Autodesk Fusion 360 part; units mm, degrees
(part 12 of 13)
move_body "Move14" bodies 13 to x (-0.996195, -0.007596, -0.086824) y (0.007596, -0.999971, 0.00033) z (-0.086824, -0.00033, 0.996224) at (0.1324, 24.9366, 0.0754)
pattern_circular "C-Pattern1" count 19 over 360 about axis through (0, 21.0013, 0) along (0, 1, 0) of bodies 11 10 12 13 makes body 14 at (9.784, 8.8123, 30.6307) makes body 15 at (19.1996, 8.8123, 25.7942) makes body 16 at (26.5347, 8.8123, 18.1625) makes body 17 at (30.9943, 8.8123, 8.5626) makes body 18 at (32.0952, 8.8123, -1.9652) makes body 19 at (30.619, 8.8187, -12.7139) makes body 20 at (24.1206, 8.8123, -21.2641) makes body 21 at (15.9092, 8.8123, -27.9439) makes body 22 at (5.9739, 8.8123, -31.5955) makes body 23 at (-4.6089, 8.8123, -31.8233) makes body 24 at (-16.9424, 10.1887, -27.2692) makes body 25 at (-23.1833, 8.8123, -22.2822) makes body 26 at (-29.1622, 8.8123, -13.5473) makes body 27 at (-31.9809, 8.8123, -3.3443) makes body 28 at (-31.334, 8.8123, 7.2211) makes body 29 at (-25.777, 10.1887, 19.1364) makes body 30 at (-18.1668, 10.1887, 26.4693) makes body 31 at (-11.0928, 8.8123, 30.1813) makes body 32 at (12.3444, 14.8255, 29.6077) makes body 33 at (21.2891, 14.8255, 23.9952) makes body 34 at (27.9268, 14.8255, 15.7825) makes body 35 at (31.5383, 14.8255, 5.8596) makes body 36 at (31.732, 14.8255, -4.6984) makes body 37 at (28.4871, 14.8255, -14.7472) makes body 38 at (22.1552, 14.8255, -23.1979) makes body 39 at (13.4224, 14.8255, -29.1348) makes body 40 at (3.2351, 14.8255, -31.9144) makes body 41 at (-7.3027, 14.8255, -31.2357) makes body 42 at (-17.0493, 14.8255, -27.172) makes body 43 at (-24.9482, 14.8255, -20.1639) makes body 44 at (-29.1662, 16.1785, -13.4098) makes body 45 at (-32.0726, 14.8255, -0.5886) makes body 46 at (-30.5259, 14.8255, 9.8572) makes body 47 at (-25.6713, 14.8255, 19.2349) makes body 48 at (-20.1593, 16.1785, 24.9818) makes body 49 at (-8.444, 14.8255, 30.9467) makes body 50 at (8.2567, 4.6533, 30.7238) makes body 51 at (17.7854, 4.6533, 26.3782) makes body 52 at (26.1953, 4.3944, 19.7024) makes body 53 at (30.237, 4.6533, 9.8921) makes body 54 at (32.7732, 4.3944, -0.5416) makes body 55 at (30.8216, 4.3944, -11.1537) makes body 56 at (24.0979, 3.4285, -21.7307) makes body 57 at (17.4719, 4.3944, -27.7329) makes body 58 at (7.3188, 3.6873, -30.6953) makes body 59 at (-3.0871, 4.6533, -31.6638) makes body 60 at (-13.2011, 4.6533, -28.9458) makes body 61 at (-21.8845, 4.6533, -23.0911) makes body 62 at (-27.9594, 3.6873, -14.6301) makes body 63 at (-31.4528, 4.6533, -4.7803) makes body 64 at (-31.9862, 3.4285, 5.8649) makes body 65 at (-27.7568, 4.6533, 15.5463) makes body 66 at (-21.205, 4.6533, 23.7166) makes body 67 at (-12.6689, 4.3944, 30.2304) makes body 68 at (9.8773, 21.2554, 30.0481) makes body 69 at (19.2453, 20.2894, 25.4259) makes body 70 at (27.2169, 20.5479, 18.3974) makes body 71 at (30.8042, 20.2894, 8.2439) makes body 72 at (31.5534, 21.2554, -2.1987) makes body 73 at (30.0454, 21.5139, -12.6328) makes body 74 at (24.5158, 20.5479, -21.8678) makes body 75 at (15.9508, 21.5139, -28.4234) makes body 76 at (5.6145, 21.2554, -31.1276) makes body 77 at (-4.8244, 20.2894, -31.5212) makes body 78 at (-15.0708, 21.5139, -28.8996) makes body 79 at (-23.8176, 20.5479, -22.6262) makes body 80 at (-29.8738, 20.5479, -13.6667) makes body 81 at (-31.7409, 20.2894, -3.0612) makes body 82 at (-31.0151, 20.2894, 7.4109) makes body 83 at (-26.7039, 21.2554, 16.9514) makes body 84 at (-20.5821, 20.5479, 25.6047) makes body 85 at (-10.7595, 20.2894, 30.0182)

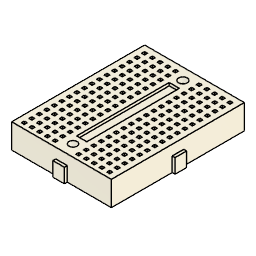
design "Mini Breadboard"
part number: 2025-09-23-19-05-31-436
Autodesk Fusion 360 part; units mm, degrees
sketch "Sketch1" plane through (0, 0, 0) normal (0, 0, 1) x (1, 0, 0)
  line L0 (17.25, 23) -> (-17.25, 23)
  line L1 (-17.25, 23) -> (-17.25, -23)
  line L2 (-17.25, -23) -> (17.25, -23)
  line L3 (17.25, -23) -> (17.25, 23)
  line L4 (17.25, 23) -> (-17.25, -23) construction
  line L5 (-17.25, 23) -> (17.25, -23) construction
  dimension "d1" = 46
  dimension "d2" = 34.5
  constraint horizontal L0
  constraint perpendicular L0 L1
  constraint parallel L0 L2
  constraint parallel L1 L3
  constraint coincident L4 origin
  constraint coincident L5 origin
  measures "d1" distance of L0.start L2.end
  measures "d2" distance of L0.start L0.end
extrude "Extrude1" add sketch "Sketch1" along normal blind 8.5
sketch "Sketch2" plane through (0, 0, 8.5) normal (0, 0, 1) x (-1, 0, 0)
  line L0 (-17.25, 23) -> (-17.25, -23)
  line L1 (-17.25, -23) -> (17.25, -23)
  line L2 (17.25, -23) -> (17.25, 23)
  line L3 (17.25, 23) -> (-17.25, 23)
  line L4 (-1.75, -16) -> (1.75, -16)
  line L5 (1.75, -16) -> (1.75, 16)
  line L6 (1.75, 16) -> (-1.75, 16)
  line L7 (-1.75, 16) -> (-1.75, -16)
  line L8 (-1.75, -16) -> (1.75, 16) construction
  line L9 (1.75, -16) -> (-1.75, 16) construction
  dimension "d5" = 32
  dimension "d6" = 3.5
  constraint horizontal L4
  constraint perpendicular L4 L5
  constraint parallel L4 L6
  constraint parallel L5 L7
  constraint coincident L8 origin
  constraint coincident L9 origin
  measures "d5" distance of L4.start L6.end
  measures "d6" distance of L4.start L4.end
extrude "Extrude2" cut sketch "Sketch2" against normal blind 1 contours L4 L5 L6 L7
sketch "Sketch3" plane through (0, 0, 8.5) normal (0, 0, 1) x (-1, 0, 0)
  line L0 (1.75, -16) -> (-1.75, -16)
  line L1 (-1.75, -16) -> (-1.75, 16)
  line L2 (-1.75, 16) -> (1.75, 16)
  line L3 (1.75, 16) -> (1.75, -16)
  line L4 (-17.25, 23) -> (-17.25, -23)
  line L5 (-17.25, -23) -> (17.25, -23)
  line L6 (17.25, -23) -> (17.25, 23)
  line L7 (17.25, 23) -> (-17.25, 23)
  line L8 (15.25, -20) -> (14.25, -20)
  line L9 (14.25, -20) -> (14.25, -21)
  line L10 (14.25, -21) -> (15.25, -21)
  line L11 (15.25, -21) -> (15.25, -20)
  line L12 (15.25, -20) -> (14.25, -21) construction
  line L13 (14.25, -20) -> (15.25, -21) construction
  point P0 (14.75, -20.5)
  dimension "d9" = 1
  dimension "d10" = 1
  dimension "d11" = 2
  dimension "d12" = 2
  constraint horizontal L8
  constraint perpendicular L8 L9
  constraint parallel L8 L10
  constraint parallel L9 L11
  constraint coincident L12 P0
  constraint coincident L13 P0
  measures "d9" distance of L9.end L10.end
  measures "d10" distance of L8.end L9.end
  measures "d11" distance of L6 L11
  measures "d12" distance of L5 L10
extrude "Extrude3" cut sketch "Sketch3" against normal blind 1 contours L8 L9 L10 L11
pattern_linear "R-Pattern1" count 5 spacing 2.67 along (1, 0, 0) count 17 spacing 2.6 along (0, -1, 0) of "Extrude3"
sketch "Sketch4" plane through (0, 0, 8.5) normal (0, 0, 1) x (-1, 0, 0)
  line L0 (3.57, 21.6) -> (4.57, 21.6)
  line L1 (4.57, 21.6) -> (4.57, 20.6)
  line L2 (4.57, 20.6) -> (3.57, 20.6)
  line L3 (3.57, 20.6) -> (3.57, 21.6)
  line L4 (6.24, 21.6) -> (7.24, 21.6)
  line L5 (7.24, 21.6) -> (7.24, 20.6)
  line L6 (7.24, 20.6) -> (6.24, 20.6)
  line L7 (6.24, 20.6) -> (6.24, 21.6)
  line L8 (8.91, 21.6) -> (9.91, 21.6)
  line L9 (9.91, 21.6) -> (9.91, 20.6)
  line L10 (9.91, 20.6) -> (8.91, 20.6)
  line L11 (8.91, 20.6) -> (8.91, 21.6)
  line L12 (11.58, 21.6) -> (12.58, 21.6)
  line L13 (12.58, 21.6) -> (12.58, 20.6)
  line L14 (12.58, 20.6) -> (11.58, 20.6)
  line L15 (11.58, 20.6) -> (11.58, 21.6)
  line L16 (14.25, 21.6) -> (15.25, 21.6)
  line L17 (15.25, 21.6) -> (15.25, 20.6)
  line L18 (15.25, 20.6) -> (14.25, 20.6)
  line L19 (14.25, 20.6) -> (14.25, 21.6)
  line L20 (3.57, 19) -> (4.57, 19)
  line L21 (4.57, 19) -> (4.57, 18)
  line L22 (4.57, 18) -> (3.57, 18)
  line L23 (3.57, 18) -> (3.57, 19)
  line L24 (6.24, 19) -> (7.24, 19)
  line L25 (7.24, 19) -> (7.24, 18)
  line L26 (7.24, 18) -> (6.24, 18)
  line L27 (6.24, 18) -> (6.24, 19)
  line L28 (8.91, 19) -> (9.91, 19)
  line L29 (9.91, 19) -> (9.91, 18)
  line L30 (9.91, 18) -> (8.91, 18)
  line L31 (8.91, 18) -> (8.91, 19)
  line L32 (11.58, 19) -> (12.58, 19)
  line L33 (12.58, 19) -> (12.58, 18)
  line L34 (12.58, 18) -> (11.58, 18)
  line L35 (11.58, 18) -> (11.58, 19)
  line L36 (14.25, 19) -> (15.25, 19)
  line L37 (15.25, 19) -> (15.25, 18)
  line L38 (15.25, 18) -> (14.25, 18)
  line L39 (14.25, 18) -> (14.25, 19)
  line L40 (3.57, 16.4) -> (4.57, 16.4)
  line L41 (4.57, 16.4) -> (4.57, 15.4)
  line L42 (4.57, 15.4) -> (3.57, 15.4)
  line L43 (3.57, 15.4) -> (3.57, 16.4)
  line L44 (6.24, 16.4) -> (7.24, 16.4)
  line L45 (7.24, 16.4) -> (7.24, 15.4)
  line L46 (7.24, 15.4) -> (6.24, 15.4)
  line L47 (6.24, 15.4) -> (6.24, 16.4)
  line L48 (8.91, 16.4) -> (9.91, 16.4)
  line L49 (9.91, 16.4) -> (9.91, 15.4)
  line L50 (9.91, 15.4) -> (8.91, 15.4)
  line L51 (8.91, 15.4) -> (8.91, 16.4)
  line L52 (11.58, 16.4) -> (12.58, 16.4)
  line L53 (12.58, 16.4) -> (12.58, 15.4)
  line L54 (12.58, 15.4) -> (11.58, 15.4)
  line L55 (11.58, 15.4) -> (11.58, 16.4)
  line L56 (14.25, 16.4) -> (15.25, 16.4)
  line L57 (15.25, 16.4) -> (15.25, 15.4)
  line L58 (15.25, 15.4) -> (14.25, 15.4)
  line L59 (14.25, 15.4) -> (14.25, 16.4)
  line L60 (3.57, 13.8) -> (4.57, 13.8)
  line L61 (4.57, 13.8) -> (4.57, 12.8)
  line L62 (4.57, 12.8) -> (3.57, 12.8)
  line L63 (3.57, 12.8) -> (3.57, 13.8)
  line L64 (6.24, 13.8) -> (7.24, 13.8)
  line L65 (7.24, 13.8) -> (7.24, 12.8)
  line L66 (7.24, 12.8) -> (6.24, 12.8)
  line L67 (6.24, 12.8) -> (6.24, 13.8)
  line L68 (8.91, 13.8) -> (9.91, 13.8)
  line L69 (9.91, 13.8) -> (9.91, 12.8)
  line L70 (9.91, 12.8) -> (8.91, 12.8)
  line L71 (8.91, 12.8) -> (8.91, 13.8)
  line L72 (11.58, 13.8) -> (12.58, 13.8)
  line L73 (12.58, 13.8) -> (12.58, 12.8)
  line L74 (12.58, 12.8) -> (11.58, 12.8)
  line L75 (11.58, 12.8) -> (11.58, 13.8)
  line L76 (14.25, 13.8) -> (15.25, 13.8)
  line L77 (15.25, 13.8) -> (15.25, 12.8)
  line L78 (15.25, 12.8) -> (14.25, 12.8)
  line L79 (14.25, 12.8) -> (14.25, 13.8)
  line L80 (3.57, 11.2) -> (4.57, 11.2)
  line L81 (4.57, 11.2) -> (4.57, 10.2)
  line L82 (4.57, 10.2) -> (3.57, 10.2)
  line L83 (3.57, 10.2) -> (3.57, 11.2)
  line L84 (6.24, 11.2) -> (7.24, 11.2)
  line L85 (7.24, 11.2) -> (7.24, 10.2)
  line L86 (7.24, 10.2) -> (6.24, 10.2)
  line L87 (6.24, 10.2) -> (6.24, 11.2)
  line L88 (8.91, 11.2) -> (9.91, 11.2)
  line L89 (9.91, 11.2) -> (9.91, 10.2)
  line L90 (9.91, 10.2) -> (8.91, 10.2)
  line L91 (8.91, 10.2) -> (8.91, 11.2)
  line L92 (11.58, 11.2) -> (12.58, 11.2)
  line L93 (12.58, 11.2) -> (12.58, 10.2)
  line L94 (12.58, 10.2) -> (11.58, 10.2)
  line L95 (11.58, 10.2) -> (11.58, 11.2)
  line L96 (14.25, 11.2) -> (15.25, 11.2)
  line L97 (15.25, 11.2) -> (15.25, 10.2)
  line L98 (15.25, 10.2) -> (14.25, 10.2)
  line L99 (14.25, 10.2) -> (14.25, 11.2)
  line L100 (3.57, 8.6) -> (4.57, 8.6)
  line L101 (4.57, 8.6) -> (4.57, 7.6)
  line L102 (4.57, 7.6) -> (3.57, 7.6)
  line L103 (3.57, 7.6) -> (3.57, 8.6)
  line L104 (6.24, 8.6) -> (7.24, 8.6)
  line L105 (7.24, 8.6) -> (7.24, 7.6)
  line L106 (7.24, 7.6) -> (6.24, 7.6)
  line L107 (6.24, 7.6) -> (6.24, 8.6)
  line L108 (8.91, 8.6) -> (9.91, 8.6)
  line L109 (9.91, 8.6) -> (9.91, 7.6)
  line L110 (9.91, 7.6) -> (8.91, 7.6)
  line L111 (8.91, 7.6) -> (8.91, 8.6)
  line L112 (11.58, 8.6) -> (12.58, 8.6)
  line L113 (12.58, 8.6) -> (12.58, 7.6)
  line L114 (12.58, 7.6) -> (11.58, 7.6)
  line L115 (11.58, 7.6) -> (11.58, 8.6)
  line L116 (14.25, 8.6) -> (15.25, 8.6)
  line L117 (15.25, 8.6) -> (15.25, 7.6)
  line L118 (15.25, 7.6) -> (14.25, 7.6)
  line L119 (14.25, 7.6) -> (14.25, 8.6)
  line L120 (3.57, 6) -> (4.57, 6)
  line L121 (4.57, 6) -> (4.57, 5)
  line L122 (4.57, 5) -> (3.57, 5)
  line L123 (3.57, 5) -> (3.57, 6)
  line L124 (6.24, 6) -> (7.24, 6)
  line L125 (7.24, 6) -> (7.24, 5)
  line L126 (7.24, 5) -> (6.24, 5)
  line L127 (6.24, 5) -> (6.24, 6)
  line L128 (8.91, 6) -> (9.91, 6)
  line L129 (9.91, 6) -> (9.91, 5)
  line L130 (9.91, 5) -> (8.91, 5)
  line L131 (8.91, 5) -> (8.91, 6)
  line L132 (11.58, 6) -> (12.58, 6)
  line L133 (12.58, 6) -> (12.58, 5)
  line L134 (12.58, 5) -> (11.58, 5)
  line L135 (11.58, 5) -> (11.58, 6)
  line L136 (14.25, 6) -> (15.25, 6)
  line L137 (15.25, 6) -> (15.25, 5)
  line L138 (15.25, 5) -> (14.25, 5)
  line L139 (14.25, 5) -> (14.25, 6)
  line L140 (3.57, 3.4) -> (4.57, 3.4)
  line L141 (4.57, 3.4) -> (4.57, 2.4)
  line L142 (4.57, 2.4) -> (3.57, 2.4)
  line L143 (3.57, 2.4) -> (3.57, 3.4)
  line L144 (6.24, 3.4) -> (7.24, 3.4)
  line L145 (7.24, 3.4) -> (7.24, 2.4)
  line L146 (7.24, 2.4) -> (6.24, 2.4)
  line L147 (6.24, 2.4) -> (6.24, 3.4)
  line L148 (8.91, 3.4) -> (9.91, 3.4)
  line L149 (9.91, 3.4) -> (9.91, 2.4)
  line L150 (9.91, 2.4) -> (8.91, 2.4)
  line L151 (8.91, 2.4) -> (8.91, 3.4)
  line L152 (11.58, 3.4) -> (12.58, 3.4)
  line L153 (12.58, 3.4) -> (12.58, 2.4)
  line L154 (12.58, 2.4) -> (11.58, 2.4)
  line L155 (11.58, 2.4) -> (11.58, 3.4)
  line L156 (14.25, 3.4) -> (15.25, 3.4)
  line L157 (15.25, 3.4) -> (15.25, 2.4)
  line L158 (15.25, 2.4) -> (14.25, 2.4)
  line L159 (14.25, 2.4) -> (14.25, 3.4)
  line L160 (3.57, 0.8) -> (4.57, 0.8)
  line L161 (4.57, 0.8) -> (4.57, -0.2)
  line L162 (4.57, -0.2) -> (3.57, -0.2)
  line L163 (3.57, -0.2) -> (3.57, 0.8)
  line L164 (6.24, 0.8) -> (7.24, 0.8)
  line L165 (7.24, 0.8) -> (7.24, -0.2)
  line L166 (7.24, -0.2) -> (6.24, -0.2)
  line L167 (6.24, -0.2) -> (6.24, 0.8)
  line L168 (8.91, 0.8) -> (9.91, 0.8)
  line L169 (9.91, 0.8) -> (9.91, -0.2)
  line L170 (9.91, -0.2) -> (8.91, -0.2)
  line L171 (8.91, -0.2) -> (8.91, 0.8)
  line L172 (11.58, 0.8) -> (12.58, 0.8)
  line L173 (12.58, 0.8) -> (12.58, -0.2)
  line L174 (12.58, -0.2) -> (11.58, -0.2)
  line L175 (11.58, -0.2) -> (11.58, 0.8)
  line L176 (14.25, 0.8) -> (15.25, 0.8)
  line L177 (15.25, 0.8) -> (15.25, -0.2)
  line L178 (15.25, -0.2) -> (14.25, -0.2)
  line L179 (14.25, -0.2) -> (14.25, 0.8)
  line L180 (3.57, -1.8) -> (4.57, -1.8)
  line L181 (4.57, -1.8) -> (4.57, -2.8)
  line L182 (4.57, -2.8) -> (3.57, -2.8)
  line L183 (3.57, -2.8) -> (3.57, -1.8)
  line L184 (6.24, -1.8) -> (7.24, -1.8)
  line L185 (7.24, -1.8) -> (7.24, -2.8)
  line L186 (7.24, -2.8) -> (6.24, -2.8)
  line L187 (6.24, -2.8) -> (6.24, -1.8)
  line L188 (8.91, -1.8) -> (9.91, -1.8)
  line L189 (9.91, -1.8) -> (9.91, -2.8)
  line L190 (9.91, -2.8) -> (8.91, -2.8)
  line L191 (8.91, -2.8) -> (8.91, -1.8)
  line L192 (11.58, -1.8) -> (12.58, -1.8)
  line L193 (12.58, -1.8) -> (12.58, -2.8)
  line L194 (12.58, -2.8) -> (11.58, -2.8)
  line L195 (11.58, -2.8) -> (11.58, -1.8)
  line L196 (14.25, -1.8) -> (15.25, -1.8)
  line L197 (15.25, -1.8) -> (15.25, -2.8)
  line L198 (15.25, -2.8) -> (14.25, -2.8)
  line L199 (14.25, -2.8) -> (14.25, -1.8)
  line L200 (3.57, -4.4) -> (4.57, -4.4)
  line L201 (4.57, -4.4) -> (4.57, -5.4)
  line L202 (4.57, -5.4) -> (3.57, -5.4)
  line L203 (3.57, -5.4) -> (3.57, -4.4)
  line L204 (6.24, -4.4) -> (7.24, -4.4)
  line L205 (7.24, -4.4) -> (7.24, -5.4)
  line L206 (7.24, -5.4) -> (6.24, -5.4)
  line L207 (6.24, -5.4) -> (6.24, -4.4)
  line L208 (8.91, -4.4) -> (9.91, -4.4)
  line L209 (9.91, -4.4) -> (9.91, -5.4)
  line L210 (9.91, -5.4) -> (8.91, -5.4)
  line L211 (8.91, -5.4) -> (8.91, -4.4)
  line L212 (11.58, -4.4) -> (12.58, -4.4)
  line L213 (12.58, -4.4) -> (12.58, -5.4)
  line L214 (12.58, -5.4) -> (11.58, -5.4)
  line L215 (11.58, -5.4) -> (11.58, -4.4)
  line L216 (14.25, -4.4) -> (15.25, -4.4)
  line L217 (15.25, -4.4) -> (15.25, -5.4)
  line L218 (15.25, -5.4) -> (14.25, -5.4)
  line L219 (14.25, -5.4) -> (14.25, -4.4)
  line L220 (3.57, -7) -> (4.57, -7)
  line L221 (4.57, -7) -> (4.57, -8)
  line L222 (4.57, -8) -> (3.57, -8)
  line L223 (3.57, -8) -> (3.57, -7)
  line L224 (6.24, -7) -> (7.24, -7)
  line L225 (7.24, -7) -> (7.24, -8)
  line L226 (7.24, -8) -> (6.24, -8)
  line L227 (6.24, -8) -> (6.24, -7)
  line L228 (8.91, -7) -> (9.91, -7)
  line L229 (9.91, -7) -> (9.91, -8)
  line L230 (9.91, -8) -> (8.91, -8)
  line L231 (8.91, -8) -> (8.91, -7)
  line L232 (11.58, -7) -> (12.58, -7)
  line L233 (12.58, -7) -> (12.58, -8)
  line L234 (12.58, -8) -> (11.58, -8)
  line L235 (11.58, -8) -> (11.58, -7)
  line L236 (14.25, -7) -> (15.25, -7)
  line L237 (15.25, -7) -> (15.25, -8)
  line L238 (15.25, -8) -> (14.25, -8)
  line L239 (14.25, -8) -> (14.25, -7)
  line L240 (3.57, -9.6) -> (4.57, -9.6)
  line L241 (4.57, -9.6) -> (4.57, -10.6)
  line L242 (4.57, -10.6) -> (3.57, -10.6)
  line L243 (3.57, -10.6) -> (3.57, -9.6)
  line L244 (6.24, -9.6) -> (7.24, -9.6)
  line L245 (7.24, -9.6) -> (7.24, -10.6)
  line L246 (7.24, -10.6) -> (6.24, -10.6)
  line L247 (6.24, -10.6) -> (6.24, -9.6)
  line L248 (8.91, -9.6) -> (9.91, -9.6)
  line L249 (9.91, -9.6) -> (9.91, -10.6)
  line L250 (9.91, -10.6) -> (8.91, -10.6)
  line L251 (8.91, -10.6) -> (8.91, -9.6)
  line L252 (11.58, -9.6) -> (12.58, -9.6)
  line L253 (12.58, -9.6) -> (12.58, -10.6)
  line L254 (12.58, -10.6) -> (11.58, -10.6)
  line L255 (11.58, -10.6) -> (11.58, -9.6)
  line L256 (14.25, -9.6) -> (15.25, -9.6)
  line L257 (15.25, -9.6) -> (15.25, -10.6)
  line L258 (15.25, -10.6) -> (14.25, -10.6)
  line L259 (14.25, -10.6) -> (14.25, -9.6)
  line L260 (3.57, -12.2) -> (4.57, -12.2)
  line L261 (4.57, -12.2) -> (4.57, -13.2)
  line L262 (4.57, -13.2) -> (3.57, -13.2)
  line L263 (3.57, -13.2) -> (3.57, -12.2)
  line L264 (6.24, -12.2) -> (7.24, -12.2)
  line L265 (7.24, -12.2) -> (7.24, -13.2)
  line L266 (7.24, -13.2) -> (6.24, -13.2)
  line L267 (6.24, -13.2) -> (6.24, -12.2)
  line L268 (8.91, -12.2) -> (9.91, -12.2)
  line L269 (9.91, -12.2) -> (9.91, -13.2)
  line L270 (9.91, -13.2) -> (8.91, -13.2)
  line L271 (8.91, -13.2) -> (8.91, -12.2)
  line L272 (11.58, -12.2) -> (12.58, -12.2)
  line L273 (12.58, -12.2) -> (12.58, -13.2)
  line L274 (12.58, -13.2) -> (11.58, -13.2)
  line L275 (11.58, -13.2) -> (11.58, -12.2)
  line L276 (14.25, -12.2) -> (15.25, -12.2)
  line L277 (15.25, -12.2) -> (15.25, -13.2)
  line L278 (15.25, -13.2) -> (14.25, -13.2)
  line L279 (14.25, -13.2) -> (14.25, -12.2)
  line L280 (3.57, -14.8) -> (4.57, -14.8)
  line L281 (4.57, -14.8) -> (4.57, -15.8)
  line L282 (4.57, -15.8) -> (3.57, -15.8)
  line L283 (3.57, -15.8) -> (3.57, -14.8)
  line L284 (6.24, -14.8) -> (7.24, -14.8)
  line L285 (7.24, -14.8) -> (7.24, -15.8)
  line L286 (7.24, -15.8) -> (6.24, -15.8)
  line L287 (6.24, -15.8) -> (6.24, -14.8)
  line L288 (8.91, -14.8) -> (9.91, -14.8)
  line L289 (9.91, -14.8) -> (9.91, -15.8)
  line L290 (9.91, -15.8) -> (8.91, -15.8)
  line L291 (8.91, -15.8) -> (8.91, -14.8)
  line L292 (11.58, -14.8) -> (12.58, -14.8)
  line L293 (12.58, -14.8) -> (12.58, -15.8)
  line L294 (12.58, -15.8) -> (11.58, -15.8)
  line L295 (11.58, -15.8) -> (11.58, -14.8)
  line L296 (14.25, -14.8) -> (15.25, -14.8)
  line L297 (15.25, -14.8) -> (15.25, -15.8)
  line L298 (15.25, -15.8) -> (14.25, -15.8)
  line L299 (14.25, -15.8) -> (14.25, -14.8)
  line L300 (3.57, -17.4) -> (4.57, -17.4)
  line L301 (4.57, -17.4) -> (4.57, -18.4)
  line L302 (4.57, -18.4) -> (3.57, -18.4)
  line L303 (3.57, -18.4) -> (3.57, -17.4)
  line L304 (6.24, -17.4) -> (7.24, -17.4)
  line L305 (7.24, -17.4) -> (7.24, -18.4)
  line L306 (7.24, -18.4) -> (6.24, -18.4)
  line L307 (6.24, -18.4) -> (6.24, -17.4)
  line L308 (8.91, -17.4) -> (9.91, -17.4)
  line L309 (9.91, -17.4) -> (9.91, -18.4)
  line L310 (9.91, -18.4) -> (8.91, -18.4)
  line L311 (8.91, -18.4) -> (8.91, -17.4)
  line L312 (11.58, -17.4) -> (12.58, -17.4)
  line L313 (12.58, -17.4) -> (12.58, -18.4)
  line L314 (12.58, -18.4) -> (11.58, -18.4)
  line L315 (11.58, -18.4) -> (11.58, -17.4)
  line L316 (14.25, -17.4) -> (15.25, -17.4)
  line L317 (15.25, -17.4) -> (15.25, -18.4)
  line L318 (15.25, -18.4) -> (14.25, -18.4)
  line L319 (14.25, -18.4) -> (14.25, -17.4)
  line L320 (3.57, -20) -> (4.57, -20)
  line L321 (4.57, -20) -> (4.57, -21)
  line L322 (4.57, -21) -> (3.57, -21)
  line L323 (3.57, -21) -> (3.57, -20)
  line L324 (6.24, -20) -> (7.24, -20)
  line L325 (7.24, -20) -> (7.24, -21)
  line L326 (7.24, -21) -> (6.24, -21)
  line L327 (6.24, -21) -> (6.24, -20)
  line L328 (8.91, -20) -> (9.91, -20)
  line L329 (9.91, -20) -> (9.91, -21)
  line L330 (9.91, -21) -> (8.91, -21)
  line L331 (8.91, -21) -> (8.91, -20)
  line L332 (11.58, -20) -> (12.58, -20)
  line L333 (12.58, -20) -> (12.58, -21)
  line L334 (12.58, -21) -> (11.58, -21)
  line L335 (11.58, -21) -> (11.58, -20)
  line L336 (14.25, -20) -> (15.25, -20)
  line L337 (15.25, -20) -> (15.25, -21)
  line L338 (15.25, -21) -> (14.25, -21)
  line L339 (14.25, -21) -> (14.25, -20)
  line L340 (1.75, -16) -> (-1.75, -16)
  line L341 (-1.75, -16) -> (-1.75, 16)
  line L342 (-1.75, 16) -> (1.75, 16)
  line L343 (1.75, 16) -> (1.75, -16)
  line L344 (-17.25, 23) -> (-17.25, -23)
  line L345 (-17.25, -23) -> (17.25, -23)
  line L346 (17.25, -23) -> (17.25, 23)
  line L347 (17.25, 23) -> (-17.25, 23)
  line L348 (-14.25, -20) -> (-15.25, -20)
  line L349 (-15.25, -20) -> (-15.25, -21)
  line L350 (-15.25, -21) -> (-14.25, -21)
  line L351 (-14.25, -21) -> (-14.25, -20)
  line L352 (-14.25, -20) -> (-15.25, -21) construction
  line L353 (-15.25, -20) -> (-14.25, -21) construction
  point P0 (-14.75, -20.5)
  dimension "d19" = 1
  dimension "d20" = 1
  dimension "d21" = 2
  dimension "d22" = 2
  constraint horizontal L348
  constraint perpendicular L348 L349
  constraint parallel L348 L350
  constraint parallel L349 L351
  constraint coincident L352 P0
  constraint coincident L353 P0
  measures "d19" distance of L348.start L348.end
  measures "d20" distance of L348.end L349.end
  measures "d21" distance of L344 L349
  measures "d22" distance of L345 L350
extrude "Extrude4" cut sketch "Sketch4" against normal blind 1 contours L348 L349 L350 L351
pattern_linear "R-Pattern2" count 5 spacing 2.67 along (-1, 0, 0) count 17 spacing 2.6 along (0, -1, 0) of "Extrude4"
sketch "Sketch5" plane through (0, 0, 8.5) normal (0, 0, 1) x (-1, 0, 0)
  line L0 (-4.57, 21.6) -> (-3.57, 21.6)
  line L1 (-3.57, 21.6) -> (-3.57, 20.6)
  line L2 (-3.57, 20.6) -> (-4.57, 20.6)
  line L3 (-4.57, 20.6) -> (-4.57, 21.6)
  line L4 (-7.24, 21.6) -> (-6.24, 21.6)
  line L5 (-6.24, 21.6) -> (-6.24, 20.6)
  line L6 (-6.24, 20.6) -> (-7.24, 20.6)
  line L7 (-7.24, 20.6) -> (-7.24, 21.6)
  line L8 (-9.91, 21.6) -> (-8.91, 21.6)
  line L9 (-8.91, 21.6) -> (-8.91, 20.6)
  line L10 (-8.91, 20.6) -> (-9.91, 20.6)
  line L11 (-9.91, 20.6) -> (-9.91, 21.6)
  line L12 (-12.58, 21.6) -> (-11.58, 21.6)
  line L13 (-11.58, 21.6) -> (-11.58, 20.6)
  line L14 (-11.58, 20.6) -> (-12.58, 20.6)
  line L15 (-12.58, 20.6) -> (-12.58, 21.6)
  line L16 (-15.25, 21.6) -> (-14.25, 21.6)
  line L17 (-14.25, 21.6) -> (-14.25, 20.6)
  line L18 (-14.25, 20.6) -> (-15.25, 20.6)
  line L19 (-15.25, 20.6) -> (-15.25, 21.6)
  line L20 (-4.57, 19) -> (-3.57, 19)
  line L21 (-3.57, 19) -> (-3.57, 18)
  line L22 (-3.57, 18) -> (-4.57, 18)
  line L23 (-4.57, 18) -> (-4.57, 19)
  line L24 (-7.24, 19) -> (-6.24, 19)
  line L25 (-6.24, 19) -> (-6.24, 18)
  line L26 (-6.24, 18) -> (-7.24, 18)
  line L27 (-7.24, 18) -> (-7.24, 19)
  line L28 (-9.91, 19) -> (-8.91, 19)
  line L29 (-8.91, 19) -> (-8.91, 18)
  line L30 (-8.91, 18) -> (-9.91, 18)
  line L31 (-9.91, 18) -> (-9.91, 19)
  line L32 (-12.58, 19) -> (-11.58, 19)
  line L33 (-11.58, 19) -> (-11.58, 18)
  line L34 (-11.58, 18) -> (-12.58, 18)
  line L35 (-12.58, 18) -> (-12.58, 19)
  line L36 (-15.25, 19) -> (-14.25, 19)
  line L37 (-14.25, 19) -> (-14.25, 18)
  line L38 (-14.25, 18) -> (-15.25, 18)
  line L39 (-15.25, 18) -> (-15.25, 19)
  line L40 (-4.57, 16.4) -> (-3.57, 16.4)
  line L41 (-3.57, 16.4) -> (-3.57, 15.4)
  line L42 (-3.57, 15.4) -> (-4.57, 15.4)
  line L43 (-4.57, 15.4) -> (-4.57, 16.4)
  line L44 (-7.24, 16.4) -> (-6.24, 16.4)
  line L45 (-6.24, 16.4) -> (-6.24, 15.4)
  line L46 (-6.24, 15.4) -> (-7.24, 15.4)
  line L47 (-7.24, 15.4) -> (-7.24, 16.4)
  line L48 (-9.91, 16.4) -> (-8.91, 16.4)
  line L49 (-8.91, 16.4) -> (-8.91, 15.4)
  line L50 (-8.91, 15.4) -> (-9.91, 15.4)
  line L51 (-9.91, 15.4) -> (-9.91, 16.4)
  line L52 (-12.58, 16.4) -> (-11.58, 16.4)
  line L53 (-11.58, 16.4) -> (-11.58, 15.4)
  line L54 (-11.58, 15.4) -> (-12.58, 15.4)
  line L55 (-12.58, 15.4) -> (-12.58, 16.4)
  line L56 (-15.25, 16.4) -> (-14.25, 16.4)
  line L57 (-14.25, 16.4) -> (-14.25, 15.4)
  line L58 (-14.25, 15.4) -> (-15.25, 15.4)
  line L59 (-15.25, 15.4) -> (-15.25, 16.4)
  line L60 (-4.57, 13.8) -> (-3.57, 13.8)
  line L61 (-3.57, 13.8) -> (-3.57, 12.8)
  line L62 (-3.57, 12.8) -> (-4.57, 12.8)
  line L63 (-4.57, 12.8) -> (-4.57, 13.8)
  line L64 (-7.24, 13.8) -> (-6.24, 13.8)
  line L65 (-6.24, 13.8) -> (-6.24, 12.8)
  line L66 (-6.24, 12.8) -> (-7.24, 12.8)
  line L67 (-7.24, 12.8) -> (-7.24, 13.8)
  line L68 (-9.91, 13.8) -> (-8.91, 13.8)
  line L69 (-8.91, 13.8) -> (-8.91, 12.8)
  line L70 (-8.91, 12.8) -> (-9.91, 12.8)
  line L71 (-9.91, 12.8) -> (-9.91, 13.8)
  line L72 (-12.58, 13.8) -> (-11.58, 13.8)
  line L73 (-11.58, 13.8) -> (-11.58, 12.8)
  line L74 (-11.58, 12.8) -> (-12.58, 12.8)
  line L75 (-12.58, 12.8) -> (-12.58, 13.8)
  line L76 (-15.25, 13.8) -> (-14.25, 13.8)
  line L77 (-14.25, 13.8) -> (-14.25, 12.8)
  line L78 (-14.25, 12.8) -> (-15.25, 12.8)
  line L79 (-15.25, 12.8) -> (-15.25, 13.8)
  line L80 (-4.57, 11.2) -> (-3.57, 11.2)
  line L81 (-3.57, 11.2) -> (-3.57, 10.2)
  line L82 (-3.57, 10.2) -> (-4.57, 10.2)
  line L83 (-4.57, 10.2) -> (-4.57, 11.2)
  line L84 (-7.24, 11.2) -> (-6.24, 11.2)
  line L85 (-6.24, 11.2) -> (-6.24, 10.2)
  line L86 (-6.24, 10.2) -> (-7.24, 10.2)
  line L87 (-7.24, 10.2) -> (-7.24, 11.2)
  line L88 (-9.91, 11.2) -> (-8.91, 11.2)
  line L89 (-8.91, 11.2) -> (-8.91, 10.2)
  line L90 (-8.91, 10.2) -> (-9.91, 10.2)
  line L91 (-9.91, 10.2) -> (-9.91, 11.2)
  line L92 (-12.58, 11.2) -> (-11.58, 11.2)
  line L93 (-11.58, 11.2) -> (-11.58, 10.2)
  line L94 (-11.58, 10.2) -> (-12.58, 10.2)
  line L95 (-12.58, 10.2) -> (-12.58, 11.2)
  line L96 (-15.25, 11.2) -> (-14.25, 11.2)
  line L97 (-14.25, 11.2) -> (-14.25, 10.2)
  line L98 (-14.25, 10.2) -> (-15.25, 10.2)
  line L99 (-15.25, 10.2) -> (-15.25, 11.2)
  line L100 (-4.57, 8.6) -> (-3.57, 8.6)
  line L101 (-3.57, 8.6) -> (-3.57, 7.6)
  line L102 (-3.57, 7.6) -> (-4.57, 7.6)
  line L103 (-4.57, 7.6) -> (-4.57, 8.6)
  line L104 (-7.24, 8.6) -> (-6.24, 8.6)
  line L105 (-6.24, 8.6) -> (-6.24, 7.6)
  line L106 (-6.24, 7.6) -> (-7.24, 7.6)
  line L107 (-7.24, 7.6) -> (-7.24, 8.6)
  line L108 (-9.91, 8.6) -> (-8.91, 8.6)
  line L109 (-8.91, 8.6) -> (-8.91, 7.6)
  line L110 (-8.91, 7.6) -> (-9.91, 7.6)
  line L111 (-9.91, 7.6) -> (-9.91, 8.6)
  line L112 (-12.58, 8.6) -> (-11.58, 8.6)
  line L113 (-11.58, 8.6) -> (-11.58, 7.6)
  line L114 (-11.58, 7.6) -> (-12.58, 7.6)
  line L115 (-12.58, 7.6) -> (-12.58, 8.6)
  line L116 (-15.25, 8.6) -> (-14.25, 8.6)
  line L117 (-14.25, 8.6) -> (-14.25, 7.6)
  line L118 (-14.25, 7.6) -> (-15.25, 7.6)
  line L119 (-15.25, 7.6) -> (-15.25, 8.6)
  line L120 (-4.57, 6) -> (-3.57, 6)
  line L121 (-3.57, 6) -> (-3.57, 5)
  line L122 (-3.57, 5) -> (-4.57, 5)
  line L123 (-4.57, 5) -> (-4.57, 6)
  line L124 (-7.24, 6) -> (-6.24, 6)
  line L125 (-6.24, 6) -> (-6.24, 5)
  line L126 (-6.24, 5) -> (-7.24, 5)
  line L127 (-7.24, 5) -> (-7.24, 6)
  line L128 (-9.91, 6) -> (-8.91, 6)
  line L129 (-8.91, 6) -> (-8.91, 5)
  line L130 (-8.91, 5) -> (-9.91, 5)
  line L131 (-9.91, 5) -> (-9.91, 6)
  line L132 (-12.58, 6) -> (-11.58, 6)
  line L133 (-11.58, 6) -> (-11.58, 5)
  line L134 (-11.58, 5) -> (-12.58, 5)
  line L135 (-12.58, 5) -> (-12.58, 6)
  line L136 (-15.25, 6) -> (-14.25, 6)
  line L137 (-14.25, 6) -> (-14.25, 5)
  line L138 (-14.25, 5) -> (-15.25, 5)
  line L139 (-15.25, 5) -> (-15.25, 6)
  line L140 (-4.57, 3.4) -> (-3.57, 3.4)
  line L141 (-3.57, 3.4) -> (-3.57, 2.4)
  line L142 (-3.57, 2.4) -> (-4.57, 2.4)
  line L143 (-4.57, 2.4) -> (-4.57, 3.4)
  line L144 (-7.24, 3.4) -> (-6.24, 3.4)
  line L145 (-6.24, 3.4) -> (-6.24, 2.4)
  line L146 (-6.24, 2.4) -> (-7.24, 2.4)
  line L147 (-7.24, 2.4) -> (-7.24, 3.4)
  line L148 (-9.91, 3.4) -> (-8.91, 3.4)
  line L149 (-8.91, 3.4) -> (-8.91, 2.4)
  line L150 (-8.91, 2.4) -> (-9.91, 2.4)
  line L151 (-9.91, 2.4) -> (-9.91, 3.4)
  line L152 (-12.58, 3.4) -> (-11.58, 3.4)
  line L153 (-11.58, 3.4) -> (-11.58, 2.4)
  line L154 (-11.58, 2.4) -> (-12.58, 2.4)
  line L155 (-12.58, 2.4) -> (-12.58, 3.4)
  line L156 (-15.25, 3.4) -> (-14.25, 3.4)
  line L157 (-14.25, 3.4) -> (-14.25, 2.4)
  line L158 (-14.25, 2.4) -> (-15.25, 2.4)
  line L159 (-15.25, 2.4) -> (-15.25, 3.4)
  line L160 (-4.57, 0.8) -> (-3.57, 0.8)
  line L161 (-3.57, 0.8) -> (-3.57, -0.2)
  line L162 (-3.57, -0.2) -> (-4.57, -0.2)
  line L163 (-4.57, -0.2) -> (-4.57, 0.8)
  line L164 (-7.24, 0.8) -> (-6.24, 0.8)
  line L165 (-6.24, 0.8) -> (-6.24, -0.2)
  line L166 (-6.24, -0.2) -> (-7.24, -0.2)
  line L167 (-7.24, -0.2) -> (-7.24, 0.8)
  line L168 (-9.91, 0.8) -> (-8.91, 0.8)
  line L169 (-8.91, 0.8) -> (-8.91, -0.2)
  line L170 (-8.91, -0.2) -> (-9.91, -0.2)
  line L171 (-9.91, -0.2) -> (-9.91, 0.8)
  line L172 (-12.58, 0.8) -> (-11.58, 0.8)
  line L173 (-11.58, 0.8) -> (-11.58, -0.2)
  line L174 (-11.58, -0.2) -> (-12.58, -0.2)
  line L175 (-12.58, -0.2) -> (-12.58, 0.8)
  line L176 (-15.25, 0.8) -> (-14.25, 0.8)
  line L177 (-14.25, 0.8) -> (-14.25, -0.2)
  line L178 (-14.25, -0.2) -> (-15.25, -0.2)
  line L179 (-15.25, -0.2) -> (-15.25, 0.8)
  line L180 (-4.57, -1.8) -> (-3.57, -1.8)
  line L181 (-3.57, -1.8) -> (-3.57, -2.8)
  line L182 (-3.57, -2.8) -> (-4.57, -2.8)
  line L183 (-4.57, -2.8) -> (-4.57, -1.8)
  line L184 (-7.24, -1.8) -> (-6.24, -1.8)
  line L185 (-6.24, -1.8) -> (-6.24, -2.8)
  line L186 (-6.24, -2.8) -> (-7.24, -2.8)
  line L187 (-7.24, -2.8) -> (-7.24, -1.8)
  line L188 (-9.91, -1.8) -> (-8.91, -1.8)
  line L189 (-8.91, -1.8) -> (-8.91, -2.8)
  line L190 (-8.91, -2.8) -> (-9.91, -2.8)
  line L191 (-9.91, -2.8) -> (-9.91, -1.8)
  line L192 (-12.58, -1.8) -> (-11.58, -1.8)
  line L193 (-11.58, -1.8) -> (-11.58, -2.8)
  line L194 (-11.58, -2.8) -> (-12.58, -2.8)
  line L195 (-12.58, -2.8) -> (-12.58, -1.8)
  line L196 (-15.25, -1.8) -> (-14.25, -1.8)
  line L197 (-14.25, -1.8) -> (-14.25, -2.8)
  line L198 (-14.25, -2.8) -> (-15.25, -2.8)
  line L199 (-15.25, -2.8) -> (-15.25, -1.8)
  line L200 (-4.57, -4.4) -> (-3.57, -4.4)
  line L201 (-3.57, -4.4) -> (-3.57, -5.4)
  line L202 (-3.57, -5.4) -> (-4.57, -5.4)
  line L203 (-4.57, -5.4) -> (-4.57, -4.4)
  line L204 (-7.24, -4.4) -> (-6.24, -4.4)
  line L205 (-6.24, -4.4) -> (-6.24, -5.4)
  line L206 (-6.24, -5.4) -> (-7.24, -5.4)
  line L207 (-7.24, -5.4) -> (-7.24, -4.4)
  line L208 (-9.91, -4.4) -> (-8.91, -4.4)
  line L209 (-8.91, -4.4) -> (-8.91, -5.4)
  line L210 (-8.91, -5.4) -> (-9.91, -5.4)
  line L211 (-9.91, -5.4) -> (-9.91, -4.4)
  line L212 (-12.58, -4.4) -> (-11.58, -4.4)
  line L213 (-11.58, -4.4) -> (-11.58, -5.4)
  line L214 (-11.58, -5.4) -> (-12.58, -5.4)
  line L215 (-12.58, -5.4) -> (-12.58, -4.4)
  line L216 (-15.25, -4.4) -> (-14.25, -4.4)
  line L217 (-14.25, -4.4) -> (-14.25, -5.4)
  line L218 (-14.25, -5.4) -> (-15.25, -5.4)
  line L219 (-15.25, -5.4) -> (-15.25, -4.4)
  line L220 (-4.57, -7) -> (-3.57, -7)
  line L221 (-3.57, -7) -> (-3.57, -8)
  line L222 (-3.57, -8) -> (-4.57, -8)
  line L223 (-4.57, -8) -> (-4.57, -7)
  line L224 (-7.24, -7) -> (-6.24, -7)
  line L225 (-6.24, -7) -> (-6.24, -8)
  line L226 (-6.24, -8) -> (-7.24, -8)
  line L227 (-7.24, -8) -> (-7.24, -7)
  line L228 (-9.91, -7) -> (-8.91, -7)
  line L229 (-8.91, -7) -> (-8.91, -8)
  line L230 (-8.91, -8) -> (-9.91, -8)
  line L231 (-9.91, -8) -> (-9.91, -7)
  line L232 (-12.58, -7) -> (-11.58, -7)
  line L233 (-11.58, -7) -> (-11.58, -8)
  line L234 (-11.58, -8) -> (-12.58, -8)
  line L235 (-12.58, -8) -> (-12.58, -7)
  line L236 (-15.25, -7) -> (-14.25, -7)
  line L237 (-14.25, -7) -> (-14.25, -8)
  line L238 (-14.25, -8) -> (-15.25, -8)
  line L239 (-15.25, -8) -> (-15.25, -7)
  line L240 (-4.57, -9.6) -> (-3.57, -9.6)
  line L241 (-3.57, -9.6) -> (-3.57, -10.6)
  line L242 (-3.57, -10.6) -> (-4.57, -10.6)
  line L243 (-4.57, -10.6) -> (-4.57, -9.6)
  line L244 (-7.24, -9.6) -> (-6.24, -9.6)
  line L245 (-6.24, -9.6) -> (-6.24, -10.6)
  line L246 (-6.24, -10.6) -> (-7.24, -10.6)
  line L247 (-7.24, -10.6) -> (-7.24, -9.6)
  line L248 (-9.91, -9.6) -> (-8.91, -9.6)
  line L249 (-8.91, -9.6) -> (-8.91, -10.6)
  line L250 (-8.91, -10.6) -> (-9.91, -10.6)
  line L251 (-9.91, -10.6) -> (-9.91, -9.6)
  line L252 (-12.58, -9.6) -> (-11.58, -9.6)
  line L253 (-11.58, -9.6) -> (-11.58, -10.6)
  line L254 (-11.58, -10.6) -> (-12.58, -10.6)
  line L255 (-12.58, -10.6) -> (-12.58, -9.6)
  line L256 (-15.25, -9.6) -> (-14.25, -9.6)
  line L257 (-14.25, -9.6) -> (-14.25, -10.6)
  line L258 (-14.25, -10.6) -> (-15.25, -10.6)
  line L259 (-15.25, -10.6) -> (-15.25, -9.6)
  line L260 (-4.57, -12.2) -> (-3.57, -12.2)
  line L261 (-3.57, -12.2) -> (-3.57, -13.2)
  line L262 (-3.57, -13.2) -> (-4.57, -13.2)
  line L263 (-4.57, -13.2) -> (-4.57, -12.2)
  line L264 (-7.24, -12.2) -> (-6.24, -12.2)
  line L265 (-6.24, -12.2) -> (-6.24, -13.2)
  line L266 (-6.24, -13.2) -> (-7.24, -13.2)
  line L267 (-7.24, -13.2) -> (-7.24, -12.2)
  line L268 (-9.91, -12.2) -> (-8.91, -12.2)
  line L269 (-8.91, -12.2) -> (-8.91, -13.2)
  line L270 (-8.91, -13.2) -> (-9.91, -13.2)
  line L271 (-9.91, -13.2) -> (-9.91, -12.2)
  line L272 (-12.58, -12.2) -> (-11.58, -12.2)
  line L273 (-11.58, -12.2) -> (-11.58, -13.2)
  line L274 (-11.58, -13.2) -> (-12.58, -13.2)
  line L275 (-12.58, -13.2) -> (-12.58, -12.2)
  line L276 (-15.25, -12.2) -> (-14.25, -12.2)
  line L277 (-14.25, -12.2) -> (-14.25, -13.2)
  line L278 (-14.25, -13.2) -> (-15.25, -13.2)
  line L279 (-15.25, -13.2) -> (-15.25, -12.2)
  line L280 (-4.57, -14.8) -> (-3.57, -14.8)
  line L281 (-3.57, -14.8) -> (-3.57, -15.8)
  line L282 (-3.57, -15.8) -> (-4.57, -15.8)
  line L283 (-4.57, -15.8) -> (-4.57, -14.8)
  line L284 (-7.24, -14.8) -> (-6.24, -14.8)
  line L285 (-6.24, -14.8) -> (-6.24, -15.8)
  line L286 (-6.24, -15.8) -> (-7.24, -15.8)
  line L287 (-7.24, -15.8) -> (-7.24, -14.8)
  line L288 (-9.91, -14.8) -> (-8.91, -14.8)
  line L289 (-8.91, -14.8) -> (-8.91, -15.8)
  line L290 (-8.91, -15.8) -> (-9.91, -15.8)
  line L291 (-9.91, -15.8) -> (-9.91, -14.8)
  line L292 (-12.58, -14.8) -> (-11.58, -14.8)
  line L293 (-11.58, -14.8) -> (-11.58, -15.8)
  line L294 (-11.58, -15.8) -> (-12.58, -15.8)
  line L295 (-12.58, -15.8) -> (-12.58, -14.8)
  line L296 (-15.25, -14.8) -> (-14.25, -14.8)
  line L297 (-14.25, -14.8) -> (-14.25, -15.8)
  line L298 (-14.25, -15.8) -> (-15.25, -15.8)
  line L299 (-15.25, -15.8) -> (-15.25, -14.8)
  line L300 (-4.57, -17.4) -> (-3.57, -17.4)
  line L301 (-3.57, -17.4) -> (-3.57, -18.4)
  line L302 (-3.57, -18.4) -> (-4.57, -18.4)
  line L303 (-4.57, -18.4) -> (-4.57, -17.4)
  line L304 (-7.24, -17.4) -> (-6.24, -17.4)
  line L305 (-6.24, -17.4) -> (-6.24, -18.4)
  line L306 (-6.24, -18.4) -> (-7.24, -18.4)
  line L307 (-7.24, -18.4) -> (-7.24, -17.4)
  line L308 (-9.91, -17.4) -> (-8.91, -17.4)
  line L309 (-8.91, -17.4) -> (-8.91, -18.4)
  line L310 (-8.91, -18.4) -> (-9.91, -18.4)
  line L311 (-9.91, -18.4) -> (-9.91, -17.4)
  line L312 (-12.58, -17.4) -> (-11.58, -17.4)
  line L313 (-11.58, -17.4) -> (-11.58, -18.4)
  line L314 (-11.58, -18.4) -> (-12.58, -18.4)
  line L315 (-12.58, -18.4) -> (-12.58, -17.4)
  line L316 (-15.25, -17.4) -> (-14.25, -17.4)
  line L317 (-14.25, -17.4) -> (-14.25, -18.4)
  line L318 (-14.25, -18.4) -> (-15.25, -18.4)
  line L319 (-15.25, -18.4) -> (-15.25, -17.4)
  line L320 (-4.57, -20) -> (-3.57, -20)
  line L321 (-3.57, -20) -> (-3.57, -21)
  line L322 (-3.57, -21) -> (-4.57, -21)
  line L323 (-4.57, -21) -> (-4.57, -20)
  line L324 (-7.24, -20) -> (-6.24, -20)
  line L325 (-6.24, -20) -> (-6.24, -21)
  line L326 (-6.24, -21) -> (-7.24, -21)
  line L327 (-7.24, -21) -> (-7.24, -20)
  line L328 (-9.91, -20) -> (-8.91, -20)
  line L329 (-8.91, -20) -> (-8.91, -21)
  line L330 (-8.91, -21) -> (-9.91, -21)
  line L331 (-9.91, -21) -> (-9.91, -20)
  line L332 (-12.58, -20) -> (-11.58, -20)
  line L333 (-11.58, -20) -> (-11.58, -21)
  line L334 (-11.58, -21) -> (-12.58, -21)
  line L335 (-12.58, -21) -> (-12.58, -20)
  line L336 (-15.25, -20) -> (-14.25, -20)
  line L337 (-14.25, -20) -> (-14.25, -21)
  line L338 (-14.25, -21) -> (-15.25, -21)
  line L339 (-15.25, -21) -> (-15.25, -20)
  line L340 (3.57, 21.6) -> (4.57, 21.6)
  line L341 (4.57, 21.6) -> (4.57, 20.6)
  line L342 (4.57, 20.6) -> (3.57, 20.6)
  line L343 (3.57, 20.6) -> (3.57, 21.6)
  line L344 (6.24, 21.6) -> (7.24, 21.6)
  line L345 (7.24, 21.6) -> (7.24, 20.6)
  line L346 (7.24, 20.6) -> (6.24, 20.6)
  line L347 (6.24, 20.6) -> (6.24, 21.6)
  line L348 (8.91, 21.6) -> (9.91, 21.6)
  line L349 (9.91, 21.6) -> (9.91, 20.6)
  line L350 (9.91, 20.6) -> (8.91, 20.6)
  line L351 (8.91, 20.6) -> (8.91, 21.6)
  line L352 (11.58, 21.6) -> (12.58, 21.6)
  line L353 (12.58, 21.6) -> (12.58, 20.6)
  line L354 (12.58, 20.6) -> (11.58, 20.6)
  line L355 (11.58, 20.6) -> (11.58, 21.6)
  line L356 (14.25, 21.6) -> (15.25, 21.6)
  line L357 (15.25, 21.6) -> (15.25, 20.6)
  line L358 (15.25, 20.6) -> (14.25, 20.6)
  line L359 (14.25, 20.6) -> (14.25, 21.6)
  line L360 (3.57, 19) -> (4.57, 19)
  line L361 (4.57, 19) -> (4.57, 18)
  line L362 (4.57, 18) -> (3.57, 18)
  line L363 (3.57, 18) -> (3.57, 19)
  line L364 (6.24, 19) -> (7.24, 19)
  line L365 (7.24, 19) -> (7.24, 18)
  line L366 (7.24, 18) -> (6.24, 18)
  line L367 (6.24, 18) -> (6.24, 19)
  line L368 (8.91, 19) -> (9.91, 19)
  line L369 (9.91, 19) -> (9.91, 18)
  line L370 (9.91, 18) -> (8.91, 18)
  line L371 (8.91, 18) -> (8.91, 19)
  line L372 (11.58, 19) -> (12.58, 19)
  line L373 (12.58, 19) -> (12.58, 18)
  line L374 (12.58, 18) -> (11.58, 18)
  line L375 (11.58, 18) -> (11.58, 19)
  line L376 (14.25, 19) -> (15.25, 19)
  line L377 (15.25, 19) -> (15.25, 18)
  line L378 (15.25, 18) -> (14.25, 18)
  line L379 (14.25, 18) -> (14.25, 19)
  line L380 (3.57, 16.4) -> (4.57, 16.4)
  line L381 (4.57, 16.4) -> (4.57, 15.4)
  line L382 (4.57, 15.4) -> (3.57, 15.4)
  line L383 (3.57, 15.4) -> (3.57, 16.4)
  line L384 (6.24, 16.4) -> (7.24, 16.4)
  line L385 (7.24, 16.4) -> (7.24, 15.4)
  line L386 (7.24, 15.4) -> (6.24, 15.4)
  line L387 (6.24, 15.4) -> (6.24, 16.4)
  line L388 (8.91, 16.4) -> (9.91, 16.4)
  line L389 (9.91, 16.4) -> (9.91, 15.4)
  line L390 (9.91, 15.4) -> (8.91, 15.4)
  line L391 (8.91, 15.4) -> (8.91, 16.4)
  line L392 (11.58, 16.4) -> (12.58, 16.4)
  line L393 (12.58, 16.4) -> (12.58, 15.4)
  line L394 (12.58, 15.4) -> (11.58, 15.4)
  line L395 (11.58, 15.4) -> (11.58, 16.4)
  line L396 (14.25, 16.4) -> (15.25, 16.4)
  line L397 (15.25, 16.4) -> (15.25, 15.4)
  line L398 (15.25, 15.4) -> (14.25, 15.4)
  line L399 (14.25, 15.4) -> (14.25, 16.4)
  line L400 (3.57, 13.8) -> (4.57, 13.8)
  line L401 (4.57, 13.8) -> (4.57, 12.8)
  line L402 (4.57, 12.8) -> (3.57, 12.8)
  line L403 (3.57, 12.8) -> (3.57, 13.8)
  line L404 (6.24, 13.8) -> (7.24, 13.8)
  line L405 (7.24, 13.8) -> (7.24, 12.8)
  line L406 (7.24, 12.8) -> (6.24, 12.8)
  line L407 (6.24, 12.8) -> (6.24, 13.8)
  line L408 (8.91, 13.8) -> (9.91, 13.8)
  line L409 (9.91, 13.8) -> (9.91, 12.8)
  line L410 (9.91, 12.8) -> (8.91, 12.8)
  line L411 (8.91, 12.8) -> (8.91, 13.8)
  line L412 (11.58, 13.8) -> (12.58, 13.8)
  line L413 (12.58, 13.8) -> (12.58, 12.8)
  line L414 (12.58, 12.8) -> (11.58, 12.8)
  line L415 (11.58, 12.8) -> (11.58, 13.8)
  line L416 (14.25, 13.8) -> (15.25, 13.8)
  line L417 (15.25, 13.8) -> (15.25, 12.8)
  line L418 (15.25, 12.8) -> (14.25, 12.8)
  line L419 (14.25, 12.8) -> (14.25, 13.8)
  line L420 (3.57, 11.2) -> (4.57, 11.2)
  line L421 (4.57, 11.2) -> (4.57, 10.2)
  line L422 (4.57, 10.2) -> (3.57, 10.2)
  line L423 (3.57, 10.2) -> (3.57, 11.2)
  line L424 (6.24, 11.2) -> (7.24, 11.2)
  line L425 (7.24, 11.2) -> (7.24, 10.2)
  line L426 (7.24, 10.2) -> (6.24, 10.2)
  line L427 (6.24, 10.2) -> (6.24, 11.2)
  line L428 (8.91, 11.2) -> (9.91, 11.2)
  line L429 (9.91, 11.2) -> (9.91, 10.2)
  line L430 (9.91, 10.2) -> (8.91, 10.2)
  line L431 (8.91, 10.2) -> (8.91, 11.2)
  line L432 (11.58, 11.2) -> (12.58, 11.2)
  line L433 (12.58, 11.2) -> (12.58, 10.2)
  line L434 (12.58, 10.2) -> (11.58, 10.2)
  line L435 (11.58, 10.2) -> (11.58, 11.2)
  line L436 (14.25, 11.2) -> (15.25, 11.2)
  line L437 (15.25, 11.2) -> (15.25, 10.2)
  line L438 (15.25, 10.2) -> (14.25, 10.2)
  line L439 (14.25, 10.2) -> (14.25, 11.2)
  line L440 (3.57, 8.6) -> (4.57, 8.6)
  line L441 (4.57, 8.6) -> (4.57, 7.6)
  line L442 (4.57, 7.6) -> (3.57, 7.6)
  line L443 (3.57, 7.6) -> (3.57, 8.6)
  line L444 (6.24, 8.6) -> (7.24, 8.6)
  line L445 (7.24, 8.6) -> (7.24, 7.6)
  line L446 (7.24, 7.6) -> (6.24, 7.6)
  line L447 (6.24, 7.6) -> (6.24, 8.6)
  line L448 (8.91, 8.6) -> (9.91, 8.6)
  line L449 (9.91, 8.6) -> (9.91, 7.6)
  line L450 (9.91, 7.6) -> (8.91, 7.6)
  line L451 (8.91, 7.6) -> (8.91, 8.6)
  line L452 (11.58, 8.6) -> (12.58, 8.6)
  line L453 (12.58, 8.6) -> (12.58, 7.6)
  line L454 (12.58, 7.6) -> (11.58, 7.6)
  line L455 (11.58, 7.6) -> (11.58, 8.6)
  line L456 (14.25, 8.6) -> (15.25, 8.6)
  line L457 (15.25, 8.6) -> (15.25, 7.6)
  line L458 (15.25, 7.6) -> (14.25, 7.6)
  line L459 (14.25, 7.6) -> (14.25, 8.6)
  line L460 (3.57, 6) -> (4.57, 6)
  line L461 (4.57, 6) -> (4.57, 5)
  line L462 (4.57, 5) -> (3.57, 5)
  line L463 (3.57, 5) -> (3.57, 6)
  line L464 (6.24, 6) -> (7.24, 6)
  line L465 (7.24, 6) -> (7.24, 5)
  line L466 (7.24, 5) -> (6.24, 5)
  line L467 (6.24, 5) -> (6.24, 6)
  line L468 (8.91, 6) -> (9.91, 6)
  line L469 (9.91, 6) -> (9.91, 5)
  line L470 (9.91, 5) -> (8.91, 5)
  line L471 (8.91, 5) -> (8.91, 6)
  line L472 (11.58, 6) -> (12.58, 6)
  line L473 (12.58, 6) -> (12.58, 5)
  line L474 (12.58, 5) -> (11.58, 5)
  line L475 (11.58, 5) -> (11.58, 6)
  line L476 (14.25, 6) -> (15.25, 6)
  line L477 (15.25, 6) -> (15.25, 5)
  line L478 (15.25, 5) -> (14.25, 5)
  line L479 (14.25, 5) -> (14.25, 6)
  line L480 (3.57, 3.4) -> (4.57, 3.4)
  line L481 (4.57, 3.4) -> (4.57, 2.4)
  line L482 (4.57, 2.4) -> (3.57, 2.4)
  line L483 (3.57, 2.4) -> (3.57, 3.4)
  line L484 (6.24, 3.4) -> (7.24, 3.4)
  line L485 (7.24, 3.4) -> (7.24, 2.4)
  line L486 (7.24, 2.4) -> (6.24, 2.4)
  line L487 (6.24, 2.4) -> (6.24, 3.4)
  line L488 (8.91, 3.4) -> (9.91, 3.4)
  line L489 (9.91, 3.4) -> (9.91, 2.4)
  line L490 (9.91, 2.4) -> (8.91, 2.4)
  line L491 (8.91, 2.4) -> (8.91, 3.4)
  line L492 (11.58, 3.4) -> (12.58, 3.4)
  line L493 (12.58, 3.4) -> (12.58, 2.4)
  line L494 (12.58, 2.4) -> (11.58, 2.4)
  line L495 (11.58, 2.4) -> (11.58, 3.4)
  line L496 (14.25, 3.4) -> (15.25, 3.4)
  line L497 (15.25, 3.4) -> (15.25, 2.4)
  line L498 (15.25, 2.4) -> (14.25, 2.4)
  line L499 (14.25, 2.4) -> (14.25, 3.4)
  line L500 (3.57, 0.8) -> (4.57, 0.8)
  line L501 (4.57, 0.8) -> (4.57, -0.2)
  line L502 (4.57, -0.2) -> (3.57, -0.2)
  line L503 (3.57, -0.2) -> (3.57, 0.8)
  line L504 (6.24, 0.8) -> (7.24, 0.8)
  line L505 (7.24, 0.8) -> (7.24, -0.2)
  line L506 (7.24, -0.2) -> (6.24, -0.2)
  line L507 (6.24, -0.2) -> (6.24, 0.8)
  line L508 (8.91, 0.8) -> (9.91, 0.8)
  line L509 (9.91, 0.8) -> (9.91, -0.2)
  line L510 (9.91, -0.2) -> (8.91, -0.2)
  line L511 (8.91, -0.2) -> (8.91, 0.8)
  line L512 (11.58, 0.8) -> (12.58, 0.8)
  line L513 (12.58, 0.8) -> (12.58, -0.2)
  line L514 (12.58, -0.2) -> (11.58, -0.2)
  line L515 (11.58, -0.2) -> (11.58, 0.8)
  line L516 (14.25, 0.8) -> (15.25, 0.8)
  line L517 (15.25, 0.8) -> (15.25, -0.2)
  line L518 (15.25, -0.2) -> (14.25, -0.2)
  line L519 (14.25, -0.2) -> (14.25, 0.8)
  line L520 (3.57, -1.8) -> (4.57, -1.8)
  line L521 (4.57, -1.8) -> (4.57, -2.8)
  line L522 (4.57, -2.8) -> (3.57, -2.8)
  line L523 (3.57, -2.8) -> (3.57, -1.8)
  line L524 (6.24, -1.8) -> (7.24, -1.8)
  line L525 (7.24, -1.8) -> (7.24, -2.8)
  line L526 (7.24, -2.8) -> (6.24, -2.8)
  line L527 (6.24, -2.8) -> (6.24, -1.8)
  line L528 (8.91, -1.8) -> (9.91, -1.8)
  line L529 (9.91, -1.8) -> (9.91, -2.8)
  line L530 (9.91, -2.8) -> (8.91, -2.8)
  line L531 (8.91, -2.8) -> (8.91, -1.8)
  line L532 (11.58, -1.8) -> (12.58, -1.8)
  line L533 (12.58, -1.8) -> (12.58, -2.8)
  line L534 (12.58, -2.8) -> (11.58, -2.8)
  line L535 (11.58, -2.8) -> (11.58, -1.8)
  line L536 (14.25, -1.8) -> (15.25, -1.8)
  line L537 (15.25, -1.8) -> (15.25, -2.8)
  line L538 (15.25, -2.8) -> (14.25, -2.8)
  line L539 (14.25, -2.8) -> (14.25, -1.8)
  line L540 (3.57, -4.4) -> (4.57, -4.4)
  line L541 (4.57, -4.4) -> (4.57, -5.4)
  line L542 (4.57, -5.4) -> (3.57, -5.4)
  line L543 (3.57, -5.4) -> (3.57, -4.4)
  line L544 (6.24, -4.4) -> (7.24, -4.4)
  line L545 (7.24, -4.4) -> (7.24, -5.4)
  line L546 (7.24, -5.4) -> (6.24, -5.4)
  line L547 (6.24, -5.4) -> (6.24, -4.4)
  line L548 (8.91, -4.4) -> (9.91, -4.4)
  line L549 (9.91, -4.4) -> (9.91, -5.4)
  line L550 (9.91, -5.4) -> (8.91, -5.4)
  line L551 (8.91, -5.4) -> (8.91, -4.4)
  line L552 (11.58, -4.4) -> (12.58, -4.4)
  line L553 (12.58, -4.4) -> (12.58, -5.4)
  line L554 (12.58, -5.4) -> (11.58, -5.4)
  line L555 (11.58, -5.4) -> (11.58, -4.4)
  line L556 (14.25, -4.4) -> (15.25, -4.4)
  line L557 (15.25, -4.4) -> (15.25, -5.4)
  line L558 (15.25, -5.4) -> (14.25, -5.4)
  line L559 (14.25, -5.4) -> (14.25, -4.4)
  line L560 (3.57, -7) -> (4.57, -7)
  line L561 (4.57, -7) -> (4.57, -8)
  line L562 (4.57, -8) -> (3.57, -8)
  line L563 (3.57, -8) -> (3.57, -7)
  line L564 (6.24, -7) -> (7.24, -7)
  line L565 (7.24, -7) -> (7.24, -8)
  line L566 (7.24, -8) -> (6.24, -8)
  line L567 (6.24, -8) -> (6.24, -7)
  line L568 (8.91, -7) -> (9.91, -7)
  line L569 (9.91, -7) -> (9.91, -8)
  line L570 (9.91, -8) -> (8.91, -8)
  line L571 (8.91, -8) -> (8.91, -7)
  line L572 (11.58, -7) -> (12.58, -7)
  line L573 (12.58, -7) -> (12.58, -8)
  line L574 (12.58, -8) -> (11.58, -8)
  line L575 (11.58, -8) -> (11.58, -7)
  line L576 (14.25, -7) -> (15.25, -7)
  line L577 (15.25, -7) -> (15.25, -8)
  line L578 (15.25, -8) -> (14.25, -8)
  line L579 (14.25, -8) -> (14.25, -7)
  line L580 (3.57, -9.6) -> (4.57, -9.6)
  line L581 (4.57, -9.6) -> (4.57, -10.6)
  line L582 (4.57, -10.6) -> (3.57, -10.6)
  line L583 (3.57, -10.6) -> (3.57, -9.6)
  line L584 (6.24, -9.6) -> (7.24, -9.6)
  line L585 (7.24, -9.6) -> (7.24, -10.6)
  line L586 (7.24, -10.6) -> (6.24, -10.6)
  line L587 (6.24, -10.6) -> (6.24, -9.6)
  line L588 (8.91, -9.6) -> (9.91, -9.6)
  line L589 (9.91, -9.6) -> (9.91, -10.6)
  line L590 (9.91, -10.6) -> (8.91, -10.6)
  line L591 (8.91, -10.6) -> (8.91, -9.6)
  line L592 (11.58, -9.6) -> (12.58, -9.6)
  line L593 (12.58, -9.6) -> (12.58, -10.6)
  line L594 (12.58, -10.6) -> (11.58, -10.6)
  line L595 (11.58, -10.6) -> (11.58, -9.6)
  line L596 (14.25, -9.6) -> (15.25, -9.6)
  line L597 (15.25, -9.6) -> (15.25, -10.6)
  line L598 (15.25, -10.6) -> (14.25, -10.6)
  line L599 (14.25, -10.6) -> (14.25, -9.6)
  line L600 (3.57, -12.2) -> (4.57, -12.2)
  line L601 (4.57, -12.2) -> (4.57, -13.2)
  line L602 (4.57, -13.2) -> (3.57, -13.2)
  line L603 (3.57, -13.2) -> (3.57, -12.2)
  line L604 (6.24, -12.2) -> (7.24, -12.2)
  line L605 (7.24, -12.2) -> (7.24, -13.2)
  line L606 (7.24, -13.2) -> (6.24, -13.2)
  line L607 (6.24, -13.2) -> (6.24, -12.2)
  line L608 (8.91, -12.2) -> (9.91, -12.2)
  line L609 (9.91, -12.2) -> (9.91, -13.2)
  line L610 (9.91, -13.2) -> (8.91, -13.2)
  line L611 (8.91, -13.2) -> (8.91, -12.2)
  line L612 (11.58, -12.2) -> (12.58, -12.2)
  line L613 (12.58, -12.2) -> (12.58, -13.2)
  line L614 (12.58, -13.2) -> (11.58, -13.2)
  line L615 (11.58, -13.2) -> (11.58, -12.2)
  line L616 (14.25, -12.2) -> (15.25, -12.2)
  line L617 (15.25, -12.2) -> (15.25, -13.2)
  line L618 (15.25, -13.2) -> (14.25, -13.2)
  line L619 (14.25, -13.2) -> (14.25, -12.2)
  line L620 (3.57, -14.8) -> (4.57, -14.8)
  line L621 (4.57, -14.8) -> (4.57, -15.8)
  line L622 (4.57, -15.8) -> (3.57, -15.8)
  line L623 (3.57, -15.8) -> (3.57, -14.8)
  line L624 (6.24, -14.8) -> (7.24, -14.8)
  line L625 (7.24, -14.8) -> (7.24, -15.8)
  line L626 (7.24, -15.8) -> (6.24, -15.8)
  line L627 (6.24, -15.8) -> (6.24, -14.8)
  line L628 (8.91, -14.8) -> (9.91, -14.8)
  line L629 (9.91, -14.8) -> (9.91, -15.8)
  line L630 (9.91, -15.8) -> (8.91, -15.8)
  line L631 (8.91, -15.8) -> (8.91, -14.8)
  line L632 (11.58, -14.8) -> (12.58, -14.8)
  line L633 (12.58, -14.8) -> (12.58, -15.8)
  line L634 (12.58, -15.8) -> (11.58, -15.8)
  line L635 (11.58, -15.8) -> (11.58, -14.8)
  line L636 (14.25, -14.8) -> (15.25, -14.8)
  line L637 (15.25, -14.8) -> (15.25, -15.8)
  line L638 (15.25, -15.8) -> (14.25, -15.8)
  line L639 (14.25, -15.8) -> (14.25, -14.8)
  line L640 (3.57, -17.4) -> (4.57, -17.4)
  line L641 (4.57, -17.4) -> (4.57, -18.4)
  line L642 (4.57, -18.4) -> (3.57, -18.4)
  line L643 (3.57, -18.4) -> (3.57, -17.4)
  line L644 (6.24, -17.4) -> (7.24, -17.4)
  line L645 (7.24, -17.4) -> (7.24, -18.4)
  line L646 (7.24, -18.4) -> (6.24, -18.4)
  line L647 (6.24, -18.4) -> (6.24, -17.4)
  line L648 (8.91, -17.4) -> (9.91, -17.4)
  line L649 (9.91, -17.4) -> (9.91, -18.4)
  line L650 (9.91, -18.4) -> (8.91, -18.4)
  line L651 (8.91, -18.4) -> (8.91, -17.4)
  line L652 (11.58, -17.4) -> (12.58, -17.4)
  line L653 (12.58, -17.4) -> (12.58, -18.4)
  line L654 (12.58, -18.4) -> (11.58, -18.4)
  line L655 (11.58, -18.4) -> (11.58, -17.4)
  line L656 (14.25, -17.4) -> (15.25, -17.4)
  line L657 (15.25, -17.4) -> (15.25, -18.4)
  line L658 (15.25, -18.4) -> (14.25, -18.4)
  line L659 (14.25, -18.4) -> (14.25, -17.4)
  line L660 (3.57, -20) -> (4.57, -20)
  line L661 (4.57, -20) -> (4.57, -21)
  line L662 (4.57, -21) -> (3.57, -21)
  line L663 (3.57, -21) -> (3.57, -20)
  line L664 (6.24, -20) -> (7.24, -20)
  line L665 (7.24, -20) -> (7.24, -21)
  line L666 (7.24, -21) -> (6.24, -21)
  line L667 (6.24, -21) -> (6.24, -20)
  line L668 (8.91, -20) -> (9.91, -20)
  line L669 (9.91, -20) -> (9.91, -21)
  line L670 (9.91, -21) -> (8.91, -21)
  line L671 (8.91, -21) -> (8.91, -20)